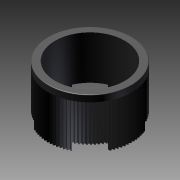
# Autodesk Inventor part: YB16SKW01-05-BBnut
Saved by Autodesk Inventor 2015 SP1 (Build 190203100, 203)
## iProperties
Category: PARTsolutions
Company: NKKSWITCHES
Created: 2013-12-31
Part Number: YB16SKW01-05-BBnut
Catalog Web Link: www.cadenas.de
Description: Panel Mount Illuminated Pushbuttons_nut-
Vendor: NKKSWITCHES
Document SubType Name: Modeling
Designer: PARTuser1
Manufacturer: NKKSWITCHES
Density: 1 g/cm^3
Material: Generic
Appearance: RGB(0.00000000000000,0.00000000000000,0.00000000000000)
PSOL_IDENT_0: {$CADENAS_DATA\23d-libs\nkkswitches\pushbuttons\yb\parts\yb_nut.prj},256 {VTYP=3D},{NB=YB16SKW01-05-
PSOL_IDENT_1: BBnut},{LINA=YB16SKW01-05-BBnut},{NN=Panel Mount Illuminated Pushbuttons_nut},{DATE=04.07.2008 12:14
PSOL_IDENT_2: :54},{GEOMDATE=04.07.2008 00:00:00},{VERSION=},{LINEID=10},{LINESUBID=-1},{WBVAR=PLS,CRCTS,PS,SHPS,C
PSOL_IDENT_3: MR,TRMNLS,LMPS,RSSTR,CTCLR}  {NB=YB16SKW01-05-BBnut},{LINA=YB16SKW01-05-BBnut},{KT=DUMMY},{PN=YB16SK
PSOL_IDENT_4: W01-05-BB},{SRS=YB},{PLS=1},{CRCTS=6},{PS=},{SHPS=S},{SHPSALG= 'S', 'S - Square (Bushing Mounting)',
PSOL_IDENT_5: 'C'  , 'C - Round (Bushing Mounting)', 'R', 'R - Rectangular (Bushing Mounting)'  , 'K', 'K - Squar
PSOL_IDENT_6: e (Snap-in Mounting)', 'M', 'M - Round (Snap-in Mounting)'  , 'N', 'N - Rectangular (Snap-in Mountin
PSOL_IDENT_7: g)' },{HSNG=K - Black only},{CMR=W},{TRMNLS=01},{A=0.709},{A1=0.591},{A11=0.827},{B=0.709},{B1=0.591
PSOL_IDENT_8: },{L=0.669},{L1=0.327},{L2=0.957},{L3=0.429},{L4=0.370},{L5=0.118},{L6=0.209},{L7=0.157},{DIA1=0.591
PSOL_IDENT_9: },{DIA=0.709},{LMPS=05},{LMPS1= '05','05 - 5-volt (Incandescent Lamp used with Solid Cap)', '12','12
PSOL_IDENT_10: - 12-volt (Incandescent Lamp used with Solid Cap)', '01','01 - 110-volt (Neon used w/ Insert Cap)',
PSOL_IDENT_11: '05','05 - 5-volt (Incandescent used w/ Insert Cap)', '12','12 - 12-volt (Incandescent used w/ Inse
PSOL_IDENT_12: rt Cap)', '5C','5C - Red (Bright LED used with LED Cap)', '5D','5D - Amber (Bright LED used with LED
PSOL_IDENT_13: Cap)', '5F','5F - Green (Bright LED used with LED Cap)', '6B','6B - White (Super Bright LED used wi
PSOL_IDENT_14: th LED Cap)', '6F','6F - Green (Super Bright LED used with LED Cap)', '6G','6G - Blue (Super Bright
PSOL_IDENT_15: LED used with LED Cap)', '1C','1C - Red Single Color (LED in Spot Illuminated Cap)', '1D','1D - Ambe
PSOL_IDENT_16: r Single Color (LED in Spot Illuminated Cap)', '1F','1F - Green Single Color (LED in Spot Illuminate
PSOL_IDENT_17: d Cap)', 'CF','CF - Red/Green Bicolor (LED in Spot Illuminated Cap)' },{RSSTR=},{RSSTR1= '','N/A' },
PSOL_IDENT_18: {CTCLR=BB},{CTCLR1= 'BB','BB - White/White (Solid Cap: Lens/Insert Colors)', 'CB','CB - Red/White (S
PSOL_IDENT_19: olid Cap: Lens/Insert Colors)', 'EB','EB - Yellow/White (Solid Cap: Lens/Insert Colors)', 'FB','FB -
PSOL_IDENT_20: Green/White (Solid Cap: Lens/Insert Colors)', 'GB','GB - Blue/White (Solid Cap: Lens/Insert Colors)
PSOL_IDENT_21: ' },{COL=0.75,0.75,0.75,0.00},{OCHR=Download pdf},{NDM=16.000}
CNS_NN: Panel Mount Illuminated Pushbuttons_nut
CNS_NB: YB16SKW01-05-BBnut
CNS_NBSYN: $PN.nut
CNS_LINA: YB16SKW01-05-BBnut
CNS_PN: YB16SKW01-05-BB
CNS_SRS: YB
CNS_PLS: 1 - SPDT
CNS_CRCTS: 6 - ON/ON
CNS_PS: Without Panel Seal
CNS_SHPS: S - Square (Bushing Mounting)
CNS_SHPSALG: 'S', 'S - Square (Bushing Mounting)', 'C'  , 'C - Round (Bushing Mounting)', 'R', 'R - Rectangular (Bushing Mounting)'  , 'K', 'K - Square (Snap-in Mounting)', 'M', 'M - Round (Snap-in Mounting)'  , 'N', 'N - Rectangular (Snap-in Mounting)'
CNS_HSNG: K - Black only
CNS_CMR: W - Silver; Rated 3A @ 125V AC
CNS_TRMNLS: 01 - Solder Lug/.110" (2.8mm) Quick Connect
CNS_A: 0.709
CNS_A1: 0.591
CNS_A11: 0.827
CNS_B: 0.709
CNS_B1: 0.591
CNS_L: 0.669
CNS_L1: 0.327
CNS_L2: 0.957
CNS_L3: 0.429
CNS_L4: 0.370
CNS_L5: 0.118
CNS_L6: 0.209
CNS_L7: 0.157
CNS_DIA1: 0.591
CNS_DIA: 0.709
CNS_LMPS: 05 - 5-volt (Incandescent Lamp for Solid Cap)
CNS_LMPS1: '05','05 - 5-volt (Incandescent Lamp used with Solid Cap)', '12','12 - 12-volt (Incandescent Lamp used with Solid Cap)', '01','01 - 110-volt (Neon used w/ Insert Cap)', '05','05 - 5-volt (Incandescent used w/ Insert Cap)', '12','12 - 12-volt (Incandescent used w/ Insert Cap)', '5C','5C - Red (Bright LED used with LED Cap)', '5D','5D - Amber (Bright LED used with LED Cap)', '5F','5F - Green (Bright LED used with LED Cap)', '6B','6B - White (Super Bright LED used with LED Cap)', '6F','6F - Green (Super Bright LED used with LED Cap)', '6G','6G - Blue (Super Bright LED used with LED Cap)', '1C','1C - Red Single Color (LED in Spot Illuminated Cap)', '1D','1D - Amber Single Color (LED in Spot Illuminated Cap)', '1F','1F - Green Single Color (LED in Spot Illuminated Cap)', 'CF','CF - Red/Green Bicolor (LED in Spot Illuminated Cap)'
CNS_RSSTR: N/A
CNS_RSSTR1: '','N/A'
CNS_CTCLR: BB - White/White (Solid Cap: Lens/Insert Colors)
CNS_CTCLR1: 'BB','BB - White/White (Solid Cap: Lens/Insert Colors)', 'CB','CB - Red/White (Solid Cap: Lens/Insert Colors)', 'EB','EB - Yellow/White (Solid Cap: Lens/Insert Colors)', 'FB','FB - Green/White (Solid Cap: Lens/Insert Colors)', 'GB','GB - Blue/White (Solid Cap: Lens/Insert Colors)'
CNS_COL: 0.75,0.75,0.75,0.00
CNS_OCHR: Download pdf
CNS_NDM: 16.000
SUPPLIER: NKKSWITCHES
ARTICLENO: YB16SKW01-05-BBnut
BOMINFO: YB16SKW01-05-BBnut
CREATOR: CADENAS GmbH
Title: YB16SKW01-05-BBnut
Author: Cadenas PARTsolutions
Autodesk Inventor part; units mm, degrees
sketch "Sketch_1" plane through (0, 0, 0) normal (0, 0, 1) x (1, 0, 0)
  line L0 (0, 0) -> (0, -10.8966)
  line L1 (0, -10.8966) -> (-8.8773, -10.8966)
  arc A0 (-9.0043, -10.7696) -> (-8.8773, -10.8966) centre (-8.8773, -10.7696) ccw
  line L2 (-9.0043, -10.7696) -> (-9.0043, -0.127)
  arc A1 (-8.8773, 0) -> (-9.0043, -0.127) centre (-8.8773, -0.127) ccw
  line L3 (-8.8773, 0) -> (0, 0)
  line L4 (0, 0) -> (0, -10.8966)
  constraints: 10 end point, 4 point on circle, 2 centre point
revolve "Revolution1" add sketch "Sketch_1" angle 360 about axis through (0, 0, 0) along (0, 1, 0)
sketch "Sketch_2" plane through (0, 0, 0) normal (0.7071068, 0, 0.7071068) x (0.7071068, 0, -0.7071068)
  line L0 (-2.7242, -10.8966) -> (2.7242, -10.8966)
  line L1 (2.7242, -10.8966) -> (2.7242, -9.398)
  line L2 (2.7242, -9.398) -> (-2.7242, -9.398)
  line L3 (-2.7242, -9.398) -> (-2.7242, -10.8966)
  constraints: 8 end point
extrude "Extrusion1" cut sketch "Sketch_2" along normal mid plane 36.0172
sketch "Sketch_3" plane through (0, 0, 0) normal (-0.7071068, 0, 0.7071068) x (0.7071068, 0, 0.7071068)
  line L0 (-2.7242, -10.8966) -> (2.7242, -10.8966)
  line L1 (2.7242, -10.8966) -> (2.7242, -9.398)
  line L2 (2.7242, -9.398) -> (-2.7242, -9.398)
  line L3 (-2.7242, -9.398) -> (-2.7242, -10.8966)
  constraints: 8 end point
extrude "Extrusion2" cut sketch "Sketch_3" along normal mid plane 36.0172
sketch "Sketch_4" plane through (0, -1.3843, 0) normal (0, 1, 0) x (1, 0, 0)
  circle A0 centre (0, 0) radius 19.05
  line L0 (-9.0043, 0) -> (-8.4911, -0.2965)
  line L1 (-8.4911, -0.2965) -> (-8.9824, -0.6281)
  line L2 (-8.9824, -0.6281) -> (-8.4498, -0.8881)
  line L3 (-8.4498, -0.8881) -> (-8.9167, -1.2532)
  line L4 (-8.9167, -1.2532) -> (-8.3672, -1.4754)
  line L5 (-8.3672, -1.4754) -> (-8.8075, -1.8721)
  line L6 (-8.8075, -1.8721) -> (-8.2439, -2.0554)
  line L7 (-8.2439, -2.0554) -> (-8.6555, -2.4819)
  line L8 (-8.6555, -2.4819) -> (-8.0805, -2.6255)
  line L9 (-8.0805, -2.6255) -> (-8.4613, -3.0797)
  line L10 (-8.4613, -3.0797) -> (-7.8776, -3.1828)
  line L11 (-7.8776, -3.1828) -> (-8.2258, -3.6624)
  line L12 (-8.2258, -3.6624) -> (-7.6364, -3.7245)
  line L13 (-7.6364, -3.7245) -> (-7.9503, -4.2273)
  line L14 (-7.9503, -4.2273) -> (-7.358, -4.2482)
  line L15 (-7.358, -4.2482) -> (-7.6361, -4.7716)
  line L16 (-7.6361, -4.7716) -> (-7.0438, -4.7511)
  line L17 (-7.0438, -4.7511) -> (-7.2846, -5.2926)
  line L18 (-7.2846, -5.2926) -> (-6.6952, -5.2308)
  line L19 (-6.6952, -5.2308) -> (-6.8977, -5.7879)
  line L20 (-6.8977, -5.7879) -> (-6.314, -5.6851)
  line L21 (-6.314, -5.6851) -> (-6.4772, -6.2549)
  line L22 (-6.4772, -6.2549) -> (-5.902, -6.1117)
  line L23 (-5.902, -6.1117) -> (-6.0251, -6.6915)
  line L24 (-6.0251, -6.6915) -> (-5.4613, -6.5085)
  line L25 (-5.4613, -6.5085) -> (-5.5436, -7.0955)
  line L26 (-5.5436, -7.0955) -> (-4.994, -6.8737)
  line L27 (-4.994, -6.8737) -> (-5.0351, -7.4649)
  line L28 (-5.0351, -7.4649) -> (-4.5024, -7.2053)
  line L29 (-4.5024, -7.2053) -> (-4.5021, -7.798)
  line L30 (-4.5021, -7.798) -> (-3.9888, -7.5018)
  line L31 (-3.9888, -7.5018) -> (-3.9472, -8.093)
  line L32 (-3.9472, -8.093) -> (-3.4558, -7.7618)
  line L33 (-3.4558, -7.7618) -> (-3.3731, -8.3486)
  line L34 (-3.3731, -8.3486) -> (-2.9059, -7.9839)
  line L35 (-2.9059, -7.9839) -> (-2.7825, -8.5636)
  line L36 (-2.7825, -8.5636) -> (-2.3419, -8.1672)
  line L37 (-2.3419, -8.1672) -> (-2.1783, -8.7368)
  line L38 (-2.1783, -8.7368) -> (-1.7665, -8.3106)
  line L39 (-1.7665, -8.3106) -> (-1.5636, -8.8675)
  line L40 (-1.5636, -8.8675) -> (-1.1825, -8.4136)
  line L41 (-1.1825, -8.4136) -> (-0.9412, -8.955)
  line L42 (-0.9412, -8.955) -> (-0.5927, -8.4756)
  line L43 (-0.5927, -8.4756) -> (-0.3142, -8.9988)
  line L44 (-0.3142, -8.9988) -> (0, -8.4963)
  line L45 (0, -8.4963) -> (0.3142, -8.9988)
  line L46 (0.3142, -8.9988) -> (0.5927, -8.4756)
  line L47 (0.5927, -8.4756) -> (0.9412, -8.955)
  line L48 (0.9412, -8.955) -> (1.1825, -8.4136)
  line L49 (1.1825, -8.4136) -> (1.5636, -8.8675)
  line L50 (1.5636, -8.8675) -> (1.7665, -8.3106)
  line L51 (1.7665, -8.3106) -> (2.1783, -8.7368)
  line L52 (2.1783, -8.7368) -> (2.3419, -8.1672)
  line L53 (2.3419, -8.1672) -> (2.7825, -8.5636)
  line L54 (2.7825, -8.5636) -> (2.9059, -7.9839)
  line L55 (2.9059, -7.9839) -> (3.3731, -8.3486)
  line L56 (3.3731, -8.3486) -> (3.4558, -7.7618)
  line L57 (3.4558, -7.7618) -> (3.9472, -8.093)
  line L58 (3.9472, -8.093) -> (3.9888, -7.5018)
  line L59 (3.9888, -7.5018) -> (4.5021, -7.798)
  line L60 (4.5021, -7.798) -> (4.5024, -7.2053)
  line L61 (4.5024, -7.2053) -> (5.0351, -7.4649)
  line L62 (5.0351, -7.4649) -> (4.994, -6.8737)
  line L63 (4.994, -6.8737) -> (5.5436, -7.0955)
  line L64 (5.5436, -7.0955) -> (5.4613, -6.5085)
  line L65 (5.4613, -6.5085) -> (6.0251, -6.6915)
  line L66 (6.0251, -6.6915) -> (5.902, -6.1117)
  line L67 (5.902, -6.1117) -> (6.4772, -6.2549)
  line L68 (6.4772, -6.2549) -> (6.314, -5.6851)
  line L69 (6.314, -5.6851) -> (6.8977, -5.7879)
  line L70 (6.8977, -5.7879) -> (6.6952, -5.2308)
  line L71 (6.6952, -5.2308) -> (7.2846, -5.2926)
  line L72 (7.2846, -5.2926) -> (7.0438, -4.7511)
  line L73 (7.0438, -4.7511) -> (7.6361, -4.7716)
  line L74 (7.6361, -4.7716) -> (7.358, -4.2482)
  line L75 (7.358, -4.2482) -> (7.9503, -4.2273)
  line L76 (7.9503, -4.2273) -> (7.6364, -3.7245)
  line L77 (7.6364, -3.7245) -> (8.2258, -3.6624)
  line L78 (8.2258, -3.6624) -> (7.8776, -3.1828)
  line L79 (7.8776, -3.1828) -> (8.4613, -3.0797)
  line L80 (8.4613, -3.0797) -> (8.0805, -2.6255)
  line L81 (8.0805, -2.6255) -> (8.6555, -2.4819)
  line L82 (8.6555, -2.4819) -> (8.2439, -2.0554)
  line L83 (8.2439, -2.0554) -> (8.8075, -1.8721)
  line L84 (8.8075, -1.8721) -> (8.3672, -1.4754)
  line L85 (8.3672, -1.4754) -> (8.9167, -1.2532)
  line L86 (8.9167, -1.2532) -> (8.4498, -0.8881)
  line L87 (8.4498, -0.8881) -> (8.9824, -0.6281)
  line L88 (8.9824, -0.6281) -> (8.4911, -0.2965)
  line L89 (8.4911, -0.2965) -> (9.0043, 0)
  line L90 (9.0043, 0) -> (8.4911, 0.2965)
  line L91 (8.4911, 0.2965) -> (8.9824, 0.6281)
  line L92 (8.9824, 0.6281) -> (8.4498, 0.8881)
  line L93 (8.4498, 0.8881) -> (8.9167, 1.2532)
  line L94 (8.9167, 1.2532) -> (8.3672, 1.4754)
  line L95 (8.3672, 1.4754) -> (8.8075, 1.8721)
  line L96 (8.8075, 1.8721) -> (8.2439, 2.0554)
  line L97 (8.2439, 2.0554) -> (8.6555, 2.4819)
  line L98 (8.6555, 2.4819) -> (8.0805, 2.6255)
  line L99 (8.0805, 2.6255) -> (8.4613, 3.0797)
  line L100 (8.4613, 3.0797) -> (7.8776, 3.1828)
  line L101 (7.8776, 3.1828) -> (8.2258, 3.6624)
  line L102 (8.2258, 3.6624) -> (7.6364, 3.7245)
  line L103 (7.6364, 3.7245) -> (7.9503, 4.2273)
  line L104 (7.9503, 4.2273) -> (7.358, 4.2482)
  line L105 (7.358, 4.2482) -> (7.6361, 4.7716)
  line L106 (7.6361, 4.7716) -> (7.0438, 4.7511)
  line L107 (7.0438, 4.7511) -> (7.2846, 5.2926)
  line L108 (7.2846, 5.2926) -> (6.6952, 5.2308)
  line L109 (6.6952, 5.2308) -> (6.8977, 5.7879)
  line L110 (6.8977, 5.7879) -> (6.314, 5.6851)
  line L111 (6.314, 5.6851) -> (6.4772, 6.2549)
  line L112 (6.4772, 6.2549) -> (5.902, 6.1117)
  line L113 (5.902, 6.1117) -> (6.0251, 6.6915)
  line L114 (6.0251, 6.6915) -> (5.4613, 6.5085)
  line L115 (5.4613, 6.5085) -> (5.5436, 7.0955)
  line L116 (5.5436, 7.0955) -> (4.994, 6.8737)
  line L117 (4.994, 6.8737) -> (5.0351, 7.4649)
  line L118 (5.0351, 7.4649) -> (4.5024, 7.2053)
  line L119 (4.5024, 7.2053) -> (4.5021, 7.798)
  line L120 (4.5021, 7.798) -> (3.9888, 7.5018)
  line L121 (3.9888, 7.5018) -> (3.9472, 8.093)
  line L122 (3.9472, 8.093) -> (3.4558, 7.7618)
  line L123 (3.4558, 7.7618) -> (3.3731, 8.3486)
  line L124 (3.3731, 8.3486) -> (2.9059, 7.9839)
  line L125 (2.9059, 7.9839) -> (2.7825, 8.5636)
  line L126 (2.7825, 8.5636) -> (2.3419, 8.1672)
  line L127 (2.3419, 8.1672) -> (2.1783, 8.7368)
  line L128 (2.1783, 8.7368) -> (1.7665, 8.3106)
  line L129 (1.7665, 8.3106) -> (1.5636, 8.8675)
  line L130 (1.5636, 8.8675) -> (1.1825, 8.4136)
  line L131 (1.1825, 8.4136) -> (0.9412, 8.955)
  line L132 (0.9412, 8.955) -> (0.5927, 8.4756)
  line L133 (0.5927, 8.4756) -> (0.3142, 8.9988)
  line L134 (0.3142, 8.9988) -> (0, 8.4963)
  line L135 (0, 8.4963) -> (-0.3142, 8.9988)
  line L136 (-0.3142, 8.9988) -> (-0.5927, 8.4756)
  line L137 (-0.5927, 8.4756) -> (-0.9412, 8.955)
  line L138 (-0.9412, 8.955) -> (-1.1825, 8.4136)
  line L139 (-1.1825, 8.4136) -> (-1.5636, 8.8675)
  line L140 (-1.5636, 8.8675) -> (-1.7665, 8.3106)
  line L141 (-1.7665, 8.3106) -> (-2.1783, 8.7368)
  line L142 (-2.1783, 8.7368) -> (-2.3419, 8.1672)
  line L143 (-2.3419, 8.1672) -> (-2.7825, 8.5636)
  line L144 (-2.7825, 8.5636) -> (-2.9059, 7.9839)
  line L145 (-2.9059, 7.9839) -> (-3.3731, 8.3486)
  line L146 (-3.3731, 8.3486) -> (-3.4558, 7.7618)
  line L147 (-3.4558, 7.7618) -> (-3.9472, 8.093)
  line L148 (-3.9472, 8.093) -> (-3.9888, 7.5018)
  line L149 (-3.9888, 7.5018) -> (-4.5021, 7.798)
  line L150 (-4.5021, 7.798) -> (-4.5024, 7.2053)
  line L151 (-4.5024, 7.2053) -> (-5.0351, 7.4649)
  line L152 (-5.0351, 7.4649) -> (-4.994, 6.8737)
  line L153 (-4.994, 6.8737) -> (-5.5436, 7.0955)
  line L154 (-5.5436, 7.0955) -> (-5.4613, 6.5085)
  line L155 (-5.4613, 6.5085) -> (-6.0251, 6.6915)
  line L156 (-6.0251, 6.6915) -> (-5.902, 6.1117)
  line L157 (-5.902, 6.1117) -> (-6.4772, 6.2549)
  line L158 (-6.4772, 6.2549) -> (-6.314, 5.6851)
  line L159 (-6.314, 5.6851) -> (-6.8977, 5.7879)
  line L160 (-6.8977, 5.7879) -> (-6.6952, 5.2308)
  line L161 (-6.6952, 5.2308) -> (-7.2846, 5.2926)
  line L162 (-7.2846, 5.2926) -> (-7.0438, 4.7511)
  line L163 (-7.0438, 4.7511) -> (-7.6361, 4.7716)
  line L164 (-7.6361, 4.7716) -> (-7.358, 4.2482)
  line L165 (-7.358, 4.2482) -> (-7.9503, 4.2273)
  line L166 (-7.9503, 4.2273) -> (-7.6364, 3.7245)
  line L167 (-7.6364, 3.7245) -> (-8.2258, 3.6624)
  line L168 (-8.2258, 3.6624) -> (-7.8776, 3.1828)
  line L169 (-7.8776, 3.1828) -> (-8.4613, 3.0797)
  line L170 (-8.4613, 3.0797) -> (-8.0805, 2.6255)
  line L171 (-8.0805, 2.6255) -> (-8.6555, 2.4819)
  line L172 (-8.6555, 2.4819) -> (-8.2439, 2.0554)
  line L173 (-8.2439, 2.0554) -> (-8.8075, 1.8721)
  line L174 (-8.8075, 1.8721) -> (-8.3672, 1.4754)
  line L175 (-8.3672, 1.4754) -> (-8.9167, 1.2532)
  line L176 (-8.9167, 1.2532) -> (-8.4498, 0.8881)
  line L177 (-8.4498, 0.8881) -> (-8.9824, 0.6281)
  line L178 (-8.9824, 0.6281) -> (-8.4911, 0.2965)
  line L179 (-8.4911, 0.2965) -> (-9.0043, 0)
  constraints: 360 end point, 1 centre point
extrude "Extrusion3" cut sketch "Sketch_4" against normal blind 18.0086
sketch "Sketch_5" plane through (0, -10.8966, 0) normal (0, 1, 0) x (1, 0, 0)
  circle A0 centre (0, 0) radius 7.5057
  constraints: 1 centre point
extrude "Extrusion4" cut sketch "Sketch_5" along normal blind 18.0086
ref_plane "nut_to_body_XY" through (0, 0, 0) normal (0, 1, 0) x (1, 0, 0)
ref_plane "nut_to_body_YZ" through (0, 0, 0) normal (1, 0, 0) x (0, 0, -1)
ref_plane "nut_to_body_ZX" through (0, 0, 0) normal (0, 0, -1) x (0, 1, 0)
body "Solid1"
